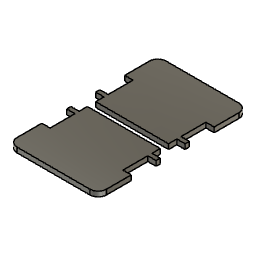
NEW Flaps design (Autodesk Fusion 360 design; units mm, degrees)
Autodesk Fusion 360 part; units mm, degrees
sketch "Sketch1" plane through (0, 0, 0) normal (0, 0, 1) x (1, 0, 0)
  line L0 (55, 190) -> (99, 190)
  arc A0 (55, 190) -> (50, 185) centre (55, 185) ccw
  arc A1 (104, 185) -> (99, 190) centre (99, 185) ccw
  line L1 (55, 147.5) -> (55, 152.5)
  line L2 (55, 152.5) -> (50, 152.5)
  line L3 (50, 155.0315) -> (55, 155.0315)
  line L4 (55, 155.0315) -> (55, 170.0315)
  line L5 (55, 170.0315) -> (50, 170.0315)
  line L6 (99, 147.5) -> (99, 152.5)
  line L7 (99, 152.5) -> (104, 152.5)
  line L8 (104, 155.031) -> (99, 155.031)
  line L9 (99, 155.031) -> (99, 170.031)
  line L10 (99, 170.031) -> (104, 170.031)
  line L11 (55, 147.5) -> (99, 147.5)
  line L12 (50, 170.0315) -> (50, 185)
  line L13 (104, 185) -> (104, 170.031)
  line L14 (104, 155.031) -> (104, 152.5)
  line L15 (50, 152.5) -> (50, 155.0315)
  line L16 (104, 105) -> (104, 119.969)
  line L17 (104, 134.969) -> (99, 134.969)
  line L18 (55, 134.9685) -> (55, 119.9685)
  line L19 (55, 142.5) -> (55, 137.5)
  line L20 (50, 134.9685) -> (55, 134.9685)
  line L21 (99, 142.5) -> (99, 137.5)
  arc A2 (99, 100) -> (104, 105) centre (99, 105) ccw
  line L22 (50, 137.5) -> (50, 134.9685)
  line L23 (50, 119.9685) -> (50, 105)
  line L24 (99, 119.969) -> (104, 119.969)
  line L25 (55, 137.5) -> (50, 137.5)
  line L26 (99, 137.5) -> (104, 137.5)
  line L27 (55, 119.9685) -> (50, 119.9685)
  line L28 (55, 100) -> (99, 100)
  line L29 (104, 134.969) -> (104, 137.5)
  arc A3 (50, 105) -> (55, 100) centre (55, 105) ccw
  line L30 (99, 134.969) -> (99, 119.969)
  line L31 (55, 142.5) -> (99, 142.5)
  point P0 (50, 190)
  point P1 (104, 190)
  point P2 (104, 100)
  point P3 (50, 100)
  dimension "d1" = 54
  dimension "d3" = 5
  dimension "d4" = 5
  constraint horizontal L0
  constraint vertical L13
  constraint coincident P0 L0
  constraint tangent L0 A0
  constraint coincident P1 L0
  constraint coincident P1 L13
  constraint tangent L0 A1
  constraint tangent A1 L13
  constraint perpendicular L3 L4
  constraint coincident L7.end L13
  constraint perpendicular L7 L13
  constraint coincident L8.start L13
  constraint perpendicular L8 L9
  constraint perpendicular L10 L13
  constraint collinear L13 L14
  measures "d1" distance of P0 P1
  measures "d3" radius of A0
  measures "d4" radius of A1
extrude "Extrude1" add sketch "Sketch1" along normal blind 3 makes body 1 at (84.3333, 113.3125, 0) makes body 2 at (84.3333, 176.6875, 0)
